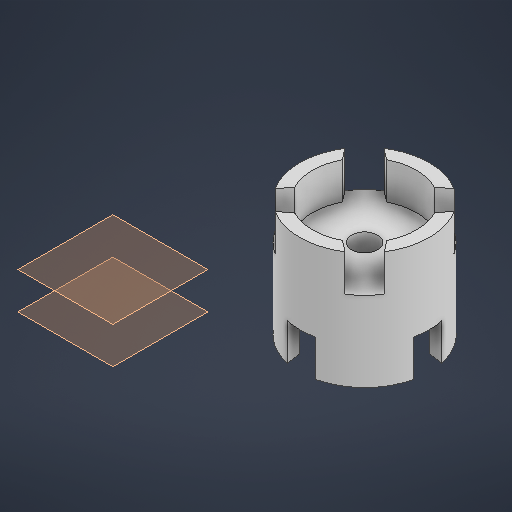
# Autodesk Inventor part: 隙間パーツ
Saved by Autodesk Inventor 2026 (Build 300175000, 175)
## iProperties
Created: 2025-10-16
Part Number: 隙間パーツ
Material: 一般
Document SubType Name: Modeling
Designer: masak
Density: 1 g/cm^3
Appearance: 既定
Author: masak
Autodesk Inventor part; units mm, degrees
ref_plane "YZ Plane" through (0, 0, 0) normal (1, 0, 0) x (0, 1, 0)
ref_plane "XZ Plane" through (0, 0, 0) normal (0, 1, 0) x (-1, 0, 0)
ref_plane "XY Plane" through (0, 0, 0) normal (0, 0, 1) x (1, 0, 0)
ref_plane "作業平面1" through (0, 8, 0) normal (0, 1, 0) x (1, 0, 0)
sketch "スケッチ2" plane through (0, 8, 0) normal (0, 1, 0) x (1, 0, 0)
  arc A0 (28.3537, 29.9285) -> (28.3537, 54.5732) centre (-4.0051, 42.2508) ccw projected
  arc A1 (39.0644, 29.9285) -> (63.709, 29.9285) centre (51.3867, 62.2873) ccw projected
  line L0 (28.3537, 29.9285) -> (39.0644, 29.9285)
  arc A2 (39.0644, 19.2178) -> (39.0644, -5.4268) centre (71.4231, 6.8955) ccw projected
  line L1 (39.0644, 29.9285) -> (39.0644, 19.2178)
  arc A3 (28.3537, -5.4268) -> (28.3537, 19.2178) centre (-4.0051, 6.8955) ccw projected
  line L2 (39.0644, 19.2178) -> (28.3537, 19.2178)
  line L3 (28.3537, 19.2178) -> (28.3537, 29.9285)
  arc A4 (3.709, 29.9285) -> (28.3537, 29.9285) centre (16.0314, 62.2873) ccw projected
  line L4 (39.0644, 29.9285) -> (28.3537, 19.2178)
  line L5 (28.3537, 29.9285) -> (39.0644, 19.2178)
  circle A5 centre (33.709, 24.5732) radius 3
  circle A6 centre (33.709, 24.5732) radius 89.9592
  circle A7 centre (33.709, 24.5732) radius 15
  circle A8 centre (33.709, 24.5732) radius 12
  line L6 (30.4879, 39.2232) -> (30.052, 36.0024)
  line L7 (19.059, 27.7943) -> (22.2798, 28.2302)
  line L8 (30.4879, 9.9231) -> (30.052, 13.144)
  circle A9 centre (33.709, 24.5732) radius 15
  circle A10 centre (33.709, 24.5732) radius 12
  line L9 (19.059, 21.352) -> (22.2798, 20.9162)
  line L10 (48.3591, 21.352) -> (45.1382, 20.9162)
  circle A11 centre (33.709, 24.5732) radius 15
  circle A12 centre (33.709, 24.5732) radius 12
  line L11 (36.9302, 9.9231) -> (37.366, 13.144)
  line L12 (36.9302, 39.2232) -> (37.366, 36.0024)
  circle A13 centre (33.709, 24.5732) radius 15
  circle A14 centre (33.709, 24.5732) radius 12
  line L13 (48.3591, 27.7943) -> (45.1382, 28.2302)
  point P0 (0, 0)
  point P1 (22.2798, 28.2302)
  point P2 (30.052, 36.0024)
  point P3 (30.4879, 39.2232)
  point P4 (19.059, 27.7943)
  point P5 (30.4879, 9.9231)
  point P6 (30.052, 13.144)
  point P7 (37.366, 13.144)
  point P8 (36.9302, 9.9231)
  point P9 (45.1382, 28.2302)
  point P10 (48.3591, 27.7943)
  dimension "d6" = 6
  dimension "d7" = 30
  dimension "d8" = 24
  dimension "d13" = 360
  constraints: 28 end point, 21 point on circle, 10 centre point, 8 coincident, 3 perpendicular, 1 horizontal, 1 midpoint, 1 point on line, 39 other
  measures "d6" diameter of A5
  measures "d7" diameter of A7
  measures "d8" diameter of A8
extrude "押し出し2" add sketch "スケッチ2" along normal blind 8.5 contours L6 A0 | A8 L7 A7 L6 | A4 L7 | L12 A7 L13 A8 | L8 A7 L9 A8 | A8 L10 A7 L11
ref_plane "作業平面2" through (0, 16.5, 0) normal (0, 1, 0) x (1, 0, 0)
sketch "スケッチ4" plane through (0, 16.5, 0) normal (0, 1, 0) x (1, 0, 0)
  arc A0 (30.052, 36.0024) -> (22.2798, 28.2302) centre (33.709, 24.5732) ccw projected
  arc A1 (28.3537, 29.9285) -> (30.052, 36.0024) centre (-4.0051, 42.2508) ccw projected
  line L0 (22.2798, 28.2302) -> (30.052, 36.0024)
  line L1 (30.052, 36.0024) -> (26.1659, 32.1163)
  arc A2 (37.366, 13.144) -> (45.1382, 20.9162) centre (33.709, 24.5732) ccw projected
  line L2 (33.709, 24.5732) -> (26.1659, 32.1163)
  circle A3 centre (33.709, 24.5732) radius 15
  point P0 (0, 0)
  constraints: 6 end point, 1 centre point, 1 coincident, 1 midpoint, 1 perpendicular
extrude "押し出し3" add sketch "スケッチ4" along normal blind 10 contours L0 A0 | A1 L2 L0 | A3
sketch "スケッチ6" plane through (33.709, 26.5, -24.5732) normal (0, 1, 0) x (1, 0, 0)
  circle A0 centre (0, 0) radius 15
  circle A1 centre (0, 0) radius 12
  arc A2 (-12.6369, -8.0814) -> (-10.6675, -5.4958) centre (-39.1679, 14.1679) ccw
  line L0 (-12.6369, -8.0814) -> (-10.6675, -5.4958)
  line L1 (-5.4958, -10.6675) -> (-8.0814, -12.6369)
  arc A3 (8.0814, -12.6369) -> (5.4958, -10.6675) centre (-14.1679, -39.1679) ccw
  line L2 (10.6675, -5.4958) -> (12.6369, -8.0814)
  arc A4 (12.6369, 8.0814) -> (10.6675, 5.4958) centre (39.1679, -14.1679) ccw
  line L3 (5.4958, 10.6675) -> (8.0814, 12.6369)
  arc A5 (-8.0814, 12.6369) -> (-5.4958, 10.6675) centre (14.1679, 39.1679) ccw
  line L4 (-10.6675, 5.4958) -> (-12.6369, 8.0814)
  point P0 (-33.709, -24.5732)
  point P1 (-10.6675, 5.4958)
  point P2 (-12.6369, 8.0814)
  point P3 (-12.6369, -8.0814)
  point P4 (-10.6675, -5.4958)
  point P5 (8.0814, -12.6369)
  point P6 (5.4958, -10.6675)
  point P7 (-5.4958, -10.6675)
  point P8 (-8.0814, -12.6369)
  point P9 (12.6369, 8.0814)
  point P10 (10.6675, 5.4958)
  point P11 (-8.0814, 12.6369)
  point P12 (-5.4958, 10.6675)
  point P13 (5.4958, 10.6675)
  dimension "d19" = 24
  dimension "d20" = 30
  dimension "d23" = 360
  constraints: 10 end point, 8 point on circle, 4 centre point, 1 coincident, 33 other
extrude "押し出し4" add sketch "スケッチ6" along normal blind 8.5 contours A0 L2 A1 A4 | L3 A1 A5 A0 | A0 L1 A1 A3 | L4 A1 L0 A0
sketch "スケッチ7" plane through (0, 16.5, 0) normal (0, -1, 0) x (1, 0, 0)
  arc A0 (44.3766, -30.0689) -> (44.3766, -19.0774) centre (33.709, -24.5732) ccw projected
  line L0 (33.709, -24.5732) -> (48.7, -24.5732)
  circle A1 centre (33.709, -24.5732) radius 3
  point P0 (0, 0)
  dimension "d27" = 6
  constraints: 2 end point, 1 centre point, 1 coincident, 1 horizontal
  measures "d27" diameter of A1
extrude "押し出し5" cut sketch "スケッチ7" against normal blind 10
